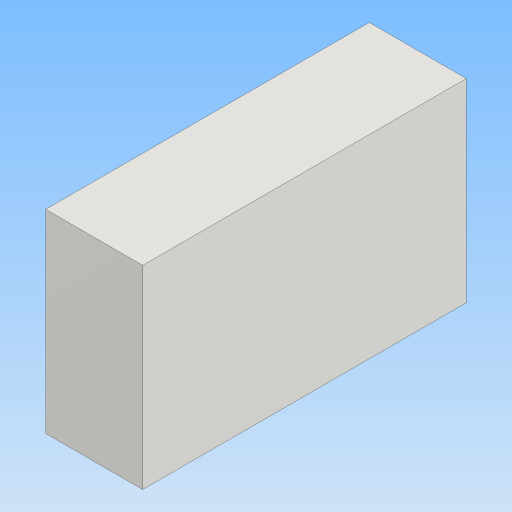
# Autodesk Inventor part: Wellennut_Rumpf_Schrauben_Block
Saved by Autodesk Inventor 2024.4 (Build 284460000, 460)
## iProperties
Created: 2026-01-22
Part Number: Wellennut_Rumpf_Schrauben_Block
Material: Generisch
Document SubType Name: Modeling
Designer: windows-desktop
Density: 1 g/cm^3
Appearance: Vorgabe
Mass: 1.44 g
Surface Area: 8.64 cm^2
Volume: 1.44 cm^3
Masse[kg]: 0,001 kg
Author: windows-desktop
Autodesk Inventor part; units mm, degrees
ref_plane "YZ Plane" through (0, 0, 0) normal (1, 0, 0) x (0, 1, 0)
ref_plane "XZ Plane" through (0, 0, 0) normal (0, 1, 0) x (-1, 0, 0)
ref_plane "XY Plane" through (0, 0, 0) normal (0, 0, 1) x (1, 0, 0)
sketch "Skizze1" plane through (0, 0, 0) normal (0, 1, 0) x (-1, 0, 0)
  line L0 (3, 6) -> (-3, 6)
  line L1 (-3, 6) -> (-3, -6)
  line L2 (-3, -6) -> (3, -6)
  line L3 (3, -6) -> (3, 6)
  line L4 (0, -8.4) -> (0, 8.4) construction
  line L5 (4.2, 0) -> (-4.2, 0) construction
  point P0 (0, 0)
  dimension "d0" = 6
  dimension "d1" = 12
  constraints: 8 end point, 2 parallel, 1 horizontal, 1 perpendicular, 2 other
  measures "d0" distance of L2.end L1.end
  measures "d1" distance of L1.end L0.end
extrude "Extrusion1" add sketch "Skizze1" along normal blind 20
